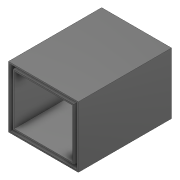
# Autodesk Inventor part: Eierkocher_final
Saved by Autodesk Inventor 2020 (Build 240168000, 168)
## iProperties
Created: 2022-02-08
Part Number: Eierkocher_final
Material: Acetalharz, Schwarz
Document SubType Name: Modeling
Designer: Julian Uhl
Density: 1.425 g/cm^3
Appearance: Glatt - Schwarz
Mass: 1111.51 g
Surface Area: 1687.5 cm^2
Volume: 780.01 cm^3
Author: Julian Uhl
Autodesk Inventor part; units mm, degrees
ref_plane "YZ Plane" through (0, 0, 0) normal (1, 0, 0) x (0, 1, 0)
ref_plane "XZ Plane" through (0, 0, 0) normal (0, 1, 0) x (-1, 0, 0)
ref_plane "XY Plane" through (0, 0, 0) normal (0, 0, 1) x (1, 0, 0)
sketch "Skizze1" plane through (0, 0, 0) normal (0, 0, 1) x (1, 0, 0)
  line L0 (-24, 0) -> (144, 0) projected
  line L1 (0, -21) -> (0, 126) projected
  line L2 (0, 0) -> (120, 0)
  line L3 (120, 0) -> (120, 105)
  line L4 (120, 105) -> (0, 105)
  line L5 (0, 105) -> (0, 0)
  line L6 (10, 10) -> (110, 10)
  line L7 (110, 10) -> (110, 95)
  line L8 (110, 95) -> (10, 95)
  line L9 (10, 95) -> (10, 10)
  dimension "d0" = 85
  dimension "d1" = 100
  dimension "d2" = 10
  dimension "d3" = 10
  dimension "d4" = 10
  dimension "d5" = 10
  constraints: 16 end point, 4 parallel, 2 horizontal, 2 perpendicular
  measures "d0" distance between parallel lines of L6 L8
  measures "d1" distance between parallel lines of L9 L7
  measures "d2" distance between parallel lines of L5 L9
  measures "d3" distance between parallel lines of L2 L6
  measures "d4" distance between parallel lines of L3 L7
  measures "d5" distance between parallel lines of L4 L8
extrude "Extrusion1" add sketch "Skizze1" along normal blind 160
sketch "Skizze2" plane through (0, 0, 0) normal (0, 0, -1) x (-1, 0, 0)
  line L0 (-120, 0) -> (-120, 105) projected
  line L1 (-120, 105) -> (0, 105) projected
  line L2 (-120, 0) -> (0, 0)
  line L3 (0, 0) -> (0, 105)
  line L4 (0, 105) -> (-120, 105)
  line L5 (-120, 105) -> (-120, 0)
  point P0 (0, 0)
  constraints: 8 end point, 2 parallel, 1 horizontal, 1 perpendicular
extrude "Extrusion2" add sketch "Skizze2" against normal blind 10
sketch "Skizze3" plane through (0, 0, 160) normal (-1, 0, 0) x (0, 0, 1)
  line L0 (-120, 95) -> (-150, 95)
  line L1 (-150, 95) -> (-150, 10)
  line L2 (-150, 10) -> (-120, 10)
  line L3 (-120, 10) -> (-120, 95)
  line L4 (-160, 105) -> (-160, 0) projected
  line L5 (-160, 0) -> (0, 0) projected
  line L6 (-160, 105) -> (0, 105) projected
  dimension "d10" = 10
  dimension "d11" = 10
  dimension "d12" = 10
  dimension "d13" = 30
  constraints: 8 end point, 2 parallel, 1 horizontal, 1 perpendicular
  measures "d10" distance between parallel lines of L4 L1
  measures "d11" distance between parallel lines of L5 L2
  measures "d12" distance between parallel lines of L6 L0
  measures "d13" distance between parallel lines of L1 L3
extrude "Extrusion3" cut sketch "Skizze3" against normal blind 10
sketch "Skizze4" plane through (0, 0, 160) normal (-1, 0, 0) x (0, 0, 1)
  line L0 (-160, 105) -> (0, 105) projected
  line L1 (-160, 0) -> (0, 0) projected
  line L2 (-100, 105) -> (-110, 105)
  line L3 (-110, 105) -> (-110, 0)
  line L4 (-110, 0) -> (-100, 0)
  line L5 (-100, 0) -> (-100, 105)
  line L6 (-120, 95) -> (-120, 10) projected
  dimension "d16" = 10
  dimension "d17" = 10
  constraints: 8 end point, 2 parallel, 2 point on line, 1 horizontal, 1 perpendicular
  measures "d16" distance between parallel lines of L3 L5
  measures "d17" distance between parallel lines of L6 L3
extrude "Extrusion4" add sketch "Skizze4" against normal blind 120
sketch "Skizze5" plane through (0, 0, 160) normal (0, 0, 1) x (1, 0, 0)
  line L0 (117.6, 102.6) -> (2.4, 102.6)
  line L1 (2.4, 102.6) -> (2.4, 2.4)
  line L2 (2.4, 2.4) -> (117.6, 2.4)
  line L3 (117.6, 2.4) -> (117.6, 102.6)
  line L4 (112.4, 97.4) -> (7.6, 97.4)
  line L5 (7.6, 97.4) -> (7.6, 7.6)
  line L6 (7.6, 7.6) -> (112.4, 7.6)
  line L7 (112.4, 7.6) -> (112.4, 97.4)
  line L8 (120, 0) -> (120, 105) projected
  line L9 (0, 0) -> (120, 0) projected
  line L10 (110, 95) -> (110, 10) projected
  line L11 (110, 10) -> (10, 10) projected
  line L12 (120, 105) -> (0, 105) projected
  line L13 (10, 95) -> (110, 95) projected
  line L14 (10, 10) -> (10, 95) projected
  line L15 (0, 105) -> (0, 0) projected
  dimension "d20" = 2.4
  dimension "d21" = 2.4
  dimension "d22" = 2.4
  dimension "d23" = 2.4
  dimension "d24" = 2.4
  dimension "d25" = 2.4
  dimension "d26" = 2.4
  dimension "d27" = 2.4
  constraints: 16 end point, 4 parallel, 2 horizontal, 2 perpendicular
  measures "d20" distance between parallel lines of L8 L3
  measures "d21" distance between parallel lines of L9 L2
  measures "d22" distance between parallel lines of L10 L7
  measures "d23" distance between parallel lines of L11 L6
  measures "d24" distance between parallel lines of L0 L12
  measures "d25" distance between parallel lines of L13 L4
  measures "d26" distance between parallel lines of L14 L5
  measures "d27" distance between parallel lines of L15 L1
extrude "Extrusion5" cut sketch "Skizze5" against normal blind 7.5 contours L3 L2 L1 L0
sketch "Skizze6" plane through (0, 0, 160) normal (-1, 0, 0) x (0, 0, 1)
  line L0 (-120, 10) -> (-120, 95) projected
  line L1 (-150, 95) -> (-150, 10) projected
  line L2 (-120, 95) -> (-150, 95)
  line L3 (-150, 95) -> (-150, 10)
  line L4 (-150, 10) -> (-120, 10)
  line L5 (-120, 10) -> (-120, 95)
  point P0 (-160, 0)
  constraints: 8 end point, 2 parallel, 1 horizontal, 1 perpendicular
extrude "Extrusion6" add sketch "Skizze6" against normal blind 10
sketch "Skizze7" plane through (0, 0, 160) normal (0, -1, 0) x (1, 0, 0)
  line L0 (10, -120) -> (110, -120)
  line L1 (110, -120) -> (110, -150)
  line L2 (110, -150) -> (10, -150)
  line L3 (10, -150) -> (10, -120)
  line L4 (0, -160) -> (120, -160) projected
  line L5 (120, -160) -> (120, 0) projected
  line L6 (0, -160) -> (0, 0) projected
  dimension "d32" = 10
  dimension "d33" = 10
  dimension "d34" = 10
  dimension "d35" = 30
  constraints: 8 end point, 2 parallel, 1 horizontal, 1 perpendicular
  measures "d32" distance between parallel lines of L4 L2
  measures "d33" distance between parallel lines of L5 L1
  measures "d34" distance between parallel lines of L6 L3
  measures "d35" distance between parallel lines of L2 L0
extrude "Extrusion7" cut sketch "Skizze7" against normal blind 10
